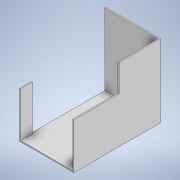
# Autodesk Inventor part: Shooting_Case
Saved by Autodesk Inventor 2020 (Build 240168000, 168)
## iProperties
Created: 2022-01-26
Part Number: Shooting_Case
Material: Generic
Document SubType Name: Modeling
Designer: danie
Density: 1 g/cm^3
Appearance: Default
Author: danie
Autodesk Inventor part; units mm, degrees
ref_plane "YZ Plane" through (0, 0, 0) normal (1, 0, 0) x (0, 1, 0)
ref_plane "XZ Plane" through (0, 0, 0) normal (0, 1, 0) x (-1, 0, 0)
ref_plane "XY Plane" through (0, 0, 0) normal (0, 0, 1) x (1, 0, 0)
sketch "Sketch1" plane through (0, 0, 0) normal (0, 1, 0) x (-1, 0, 0)
  line L0 (0, 0) -> (-146.05, 0)
  line L1 (-146.05, 0) -> (-146.05, -231.775)
  line L2 (-146.05, -231.775) -> (0, -231.775)
  line L3 (0, -231.775) -> (0, 0)
  dimension "d0" = 146.05
  dimension "d1" = 231.775
  constraints: 8 end point, 2 parallel, 1 horizontal, 1 perpendicular
  measures "d0" distance of L2.end L1.end
  measures "d1" distance of L1.end L0.end
extrude "Extrusion1" add sketch "Sketch1" along normal blind 3.175
sketch "Sketch2" plane through (146.05, 0, 0) normal (1, 0, 0) x (0, 0, -1)
  line L0 (0, 0) -> (231.775, 0) projected
  line L1 (231.775, 0) -> (231.775, 194.818)
  line L2 (231.775, 194.818) -> (120.65, 194.818)
  line L3 (120.65, 194.818) -> (120.65, 122.809)
  line L4 (0, 0) -> (0, 122.809)
  line L5 (0, 122.809) -> (120.65, 122.809)
  dimension "d4" = 194.818
  dimension "d5" = 111.125
  dimension "d6" = 72.009
  dimension "d7" = 122.809
  constraints: 10 end point, 3 vertical, 1 horizontal
  measures "d4" distance of L0.end L1.end
  measures "d5" distance of L1.end L2.end
  measures "d6" distance of L2.end L3.end
  measures "d7" distance of L0.start L4.end
extrude "Extrusion2" add sketch "Sketch2" against normal blind 3.175
sketch "Sketch3" plane through (146.05, 0, -231.775) normal (0, 0, -1) x (-1, 0, 0)
  line L0 (0, 0) -> (0, 194.818) projected
  line L1 (0, 194.818) -> (146.05, 194.818)
  line L2 (146.05, 194.818) -> (146.05, 0)
  line L3 (146.05, 0) -> (0, 0)
  line L4 (0, 0) -> (0, 194.818)
  constraints: 8 end point, 2 parallel, 1 horizontal, 1 perpendicular
extrude "Extrusion3" add sketch "Sketch3" against normal blind 3.175
sketch "Sketch4" plane through (0, 0, -231.775) normal (-1, 0, 0) x (0, 0, 1)
  line L0 (231.775, 0) -> (231.775, 3.175) projected
  line L1 (231.775, 122.809) -> (111.125, 122.809) projected
  line L2 (231.775, 0) -> (200.025, 0)
  line L3 (200.025, 0) -> (200.025, 122.809)
  line L4 (200.025, 122.809) -> (231.775, 122.809)
  line L5 (231.775, 122.809) -> (231.775, 0)
  dimension "d12" = 31.75
  constraints: 8 end point, 2 parallel, 1 horizontal, 1 perpendicular, 1 point on line
  measures "d12" distance of L3.end L4.end
extrude "Extrusion4" add sketch "Sketch4" against normal blind 3.175
body "Solid1"
